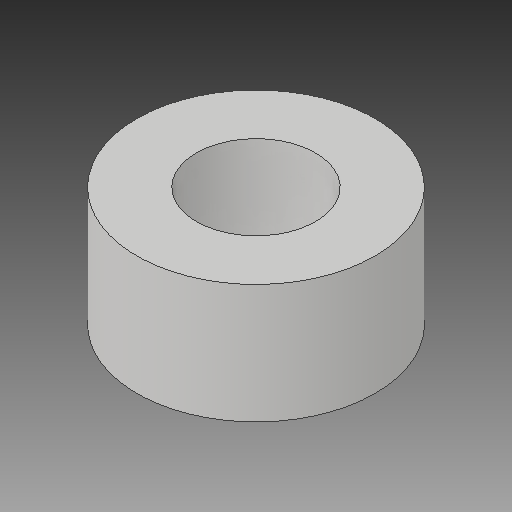
# Autodesk Inventor part: gauge_ring
Saved by Autodesk Inventor 2018 (Build 220112000, 112)
## iProperties
Created: 2018-05-01
Part Number: gauge_ring
Material: Generic
Document SubType Name: Modeling
Designer: medrimonia
Density: 1 g/cm^3
Appearance: Default
Vendor: ???
Mass: 0.150796 g
Surface Area: 2.26195 cm^2
Volume: 0.150796 cm^3
Author: medrimonia
Autodesk Inventor part; units mm, degrees
ref_plane "YZ Plane" through (0, 0, 0) normal (1, 0, 0) x (0, 1, 0)
ref_plane "XZ Plane" through (0, 0, 0) normal (0, 1, 0) x (-1, 0, 0)
ref_plane "XY Plane" through (0, 0, 0) normal (0, 0, 1) x (1, 0, 0)
sketch "Sketch1" plane through (0, 0, 0) normal (0, 1, 0) x (-1, 0, 0)
  circle A0 centre (0, 0) radius 2
  circle A1 centre (0, 0) radius 4
  dimension "d0" = 4
  dimension "d1" = 8
  constraints: 2 centre point, 2 coincident
  measures "d0" diameter of A0
  measures "d1" diameter of A1
extrude "Extrusion1" add sketch "Sketch1" along normal blind 4
equation "\"d0\" = hole_diameter"
equation "\"d1\" = ring_diameter"
equation "\"d2\" = ring_height"
equation "\"hole_diameter\" = 4"
equation "\"ring_diameter\" = 8"
equation "\"ring_height\" = 4"
body "Solid1"
